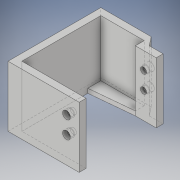
# Autodesk Inventor part: Swivel Arm Servo Holder
Saved by Autodesk Inventor 2019 (Build 230136000, 136)
## iProperties
Created: 2020-04-05
Part Number: Swivel Arm Servo Holder
Material: Generic
Document SubType Name: Modeling
Designer: isaac
Density: 1 g/cm^3
Appearance: Default
Author: isaac
Autodesk Inventor part; units mm, degrees
ref_plane "YZ Plane" through (0, 0, 0) normal (1, 0, 0) x (0, 1, 0)
ref_plane "XZ Plane" through (0, 0, 0) normal (0, 1, 0) x (-1, 0, 0)
ref_plane "XY Plane" through (0, 0, 0) normal (0, 0, 1) x (1, 0, 0)
sketch "Sketch14" plane through (0, 0, 0) normal (0, 1, 0) x (-1, 0, 0)
  line L0 (0, 0) -> (0, -45.5)
  line L1 (0, -45.5) -> (-25, -45.5)
  line L2 (-25, -45.5) -> (-25, -40.4)
  line L3 (-25, -40.4) -> (-37, -40.4)
  line L4 (-33, 0) -> (0, 0)
  line L5 (0, 4) -> (4, 4)
  line L6 (4, 4) -> (4, -45.5)
  line L7 (4, -45.5) -> (4, -49.5)
  line L8 (4, -49.5) -> (-25, -49.5)
  line L9 (-37, -40.4) -> (-37, -44.4)
  line L10 (-33, 0) -> (-37, 0)
  line L11 (-37, 0) -> (-37, 4)
  line L12 (-37, 4) -> (0, 4)
  line L13 (-37, -44.4) -> (-29, -44.4)
  line L14 (-29, -44.4) -> (-25, -49.5)
  dimension "d59" = 45.5
  dimension "d60" = 25
  dimension "d61" = 5.1
  dimension "d62" = 12
  dimension "d64" = 4
  dimension "d65" = 4
  dimension "d66" = 4
  dimension "d67" = 4
  dimension "d68" = 8
  constraints: 30 end point, 6 perpendicular, 3 horizontal, 3 vertical, 1 point on line
  measures "d59" distance of L0.start L0.end
  measures "d60" distance of L0.end L1.end
  measures "d61" distance of L1.end L2.end
  measures "d62" distance of L2.end L3.end
  measures "d64" distance of L5.start L5.end
  measures "d65" distance of L6.end L7.end
  measures "d66" distance of L3.end L9.end
  measures "d67" distance between parallel lines of L4 L12
  measures "d68" distance of L9.end L13.end
extrude "Extrusion10" add sketch "Sketch14" along normal blind 35
sketch "Sketch17" plane through (0, 0, 0) normal (0, -1, 0) x (1, 0, 0)
  line L0 (0, -37.9754) -> (25, -40.4) projected
  line L1 (0, 0) -> (0, -45.5) projected
  line L2 (0, -37.9754) -> (0, -45.5)
  line L3 (25, -45.5) -> (0, -45.5) projected
  line L4 (0, -45.5) -> (25, -45.5)
  line L5 (25, -45.5) -> (25, -40.4) projected
  line L6 (25, -45.5) -> (25, -40.4)
  line L7 (25, -40.4) -> (0, -37.9754)
  constraints: 8 end point, 3 collinear
extrude "Extrusion12" add sketch "Sketch17" against normal blind 2.5
sketch "Sketch18" plane through (25, 0, -49.5) normal (0, 0, -1) x (-1, 0, 0)
  line L0 (25, 2.5) -> (25, 35) projected
  line L1 (25, 35) -> (-4.7, 35) construction
  line L2 (-4.7, 35) -> (-4.7, 15) construction
  line L3 (-4.7, 15) -> (25, 15) construction
  line L4 (25, 15) -> (25, 35) construction
  point P0 (25, 0)
  point P1 (-4.7, 25)
  dimension "d77" = 29.7
  dimension "d78" = 20
  constraints: 8 end point, 2 parallel, 1 coincident, 1 horizontal, 1 midpoint, 1 perpendicular
  measures "d77" distance of L3.end L2.end
  measures "d78" distance of L2.end L1.end
hole "Hole4" at (29.7, 15, -49.5) at (29.7, 25, -49.5) direction (0, 0, 1) diameter 3.5 depth 9.1 counterbore diameter 4.5 counterbore depth 7.6
sketch "Sketch19" plane through (-4, 0, 4) normal (0, 0, 1) x (1, 0, 0)
  circle A0 centre (33.7, 25) radius 1.75 projected
  circle A1 centre (33.7, 15) radius 1.75 projected
  point P0 (4, 0)
  constraints: 2 coincident
hole "Hole5" at (29.7, 25, 4) at (29.7, 15, 4) direction (0, 0, -1) diameter 3.5 depth 4 counterbore diameter 4.5 counterbore depth 2.5
body "Solid2"
